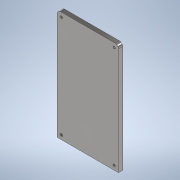
# Autodesk Inventor part: backdor
Saved by Autodesk Inventor 2021 (Build 250183000, 183)
## iProperties
Created: 2023-04-06
Part Number: backdor
Material: Steel
Document SubType Name: Modeling
Designer: EF0481
Density: 7.85 g/cm^3
Appearance: Steel - Polished
Author: EF0481
Autodesk Inventor part; units mm, degrees
ref_plane "YZ Plane" through (0, 0, 0) normal (1, 0, 0) x (0, 1, 0)
ref_plane "XZ Plane" through (0, 0, 0) normal (0, 1, 0) x (-1, 0, 0)
ref_plane "XY Plane" through (0, 0, 0) normal (0, 0, 1) x (1, 0, 0)
sketch "Sketch1" plane through (0, 0, 0) normal (0, 0, 1) x (1, 0, 0)
  line L0 (0, 0) -> (72, 0)
  line L1 (72, 0) -> (72, 130)
  line L2 (72, 130) -> (0, 130)
  line L3 (0, 130) -> (0, 0)
  dimension "d0" = 72
  dimension "d1" = 130
  constraints: 8 end point, 2 parallel, 1 horizontal, 1 perpendicular
  measures "d0" distance of L2.end L1.end
  measures "d1" distance of L1.end L0.end
extrude "Extrusion1" add sketch "Sketch1" against normal blind 5
fillet "Fillet1" radius 4 1 edges at (72, 130, -2.5)
fillet "Fillet2" radius 4 1 edges at (0, 130, -2.5)
sketch "Sketch2" plane through (0, 0, -5) normal (0, 0, -1) x (-1, 0, 0)
  circle A0 centre (-67, 125) radius 1.5
  line L0 (-72, 126) -> (-72, 0) projected
  line L1 (-4, 130) -> (-68, 130) projected
  line L2 (0, 0) -> (0, 126) projected
  arc A1 (0, 126) -> (-4, 130) centre (-4, 126) ccw projected
  line L3 (-4, 130) -> (-68, 130) projected
  arc A2 (-68, 130) -> (-72, 126) centre (-68, 126) ccw projected
  line L4 (-72, 126) -> (-72, 0) projected
  line L5 (-72, 0) -> (0, 0) projected
  line L6 (0, 0) -> (0, 126) projected
  line L7 (-68, 130) -> (-4, 130) projected
  line L8 (0, 0) -> (-72, 0) projected
  circle A3 centre (-5, 125) radius 1.5
  circle A4 centre (-67, 5) radius 1.5
  line L9 (-36, 130) -> (-36, 0)
  circle A5 centre (-5, 5) radius 1.5
  dimension "d7" = 3
  dimension "d8" = 5
  dimension "d9" = 5
  dimension "d10" = 3
  dimension "d11" = 5
  dimension "d12" = 5
  constraints: 4 centre point, 2 end point, 2 midpoint, 1 symmetric about line, 1 other
  measures "d7" diameter of A0
  measures "d8" distance from line of L0 A0.centre
  measures "d9" distance from line of L1 A0.centre
  measures "d10" diameter of A4
  measures "d11" distance from line of A4.centre L0
  measures "d12" distance from line of L5 A4.centre
hole "Hole1" at (67, 125, -5) at (5, 125, -5) at (67, 5, -5) at (5, 5, -5) direction (0, 0, 1) diameter 2.6416 depth 10.979 thread size "6-32 UNC" class "2B" standard "ANSI Unified Screw Threads"
body "Solid1"
